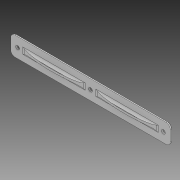
# Autodesk Inventor part: LEDLid
Saved by Autodesk Inventor 2020 (Build 240168000, 168)
## iProperties
Created: 2020-12-20
Part Number: LEDLid
Material: Generic
Document SubType Name: Modeling
Designer: DDeGo
Density: 1 g/cm^3
Appearance: Default
Author: DDeGo
Autodesk Inventor part; units mm, degrees
ref_plane "YZ Plane" through (0, 0, 0) normal (1, 0, 0) x (0, 1, 0)
ref_plane "XZ Plane" through (0, 0, 0) normal (0, 1, 0) x (-1, 0, 0)
ref_plane "XY Plane" through (0, 0, 0) normal (0, 0, 1) x (1, 0, 0)
sketch "Sketch1" plane through (0, 0, 0) normal (0, 0, 1) x (1, 0, 0)
  line L0 (71, -9) -> (-71, -9)
  line L1 (-75, -5) -> (-75, 5)
  line L2 (-71, 9) -> (71, 9)
  line L3 (75, 5) -> (75, -5)
  line L4 (75, -9) -> (-75, 9) construction
  line L5 (-75, -9) -> (75, 9) construction
  arc A0 (-71, 9) -> (-75, 5) centre (-71, 5) ccw
  arc A1 (-75, -5) -> (-71, -9) centre (-71, -5) ccw
  arc A2 (75, 5) -> (71, 9) centre (71, 5) ccw
  arc A3 (71, -9) -> (75, -5) centre (71, -5) ccw
  circle A4 centre (0, 0) radius 1.75
  line L6 (-75, 0) -> (-68.5, 0) construction
  line L7 (75, 0) -> (68.5, 0) construction
  circle A5 centre (-68.5, 0) radius 1.75
  circle A6 centre (68.5, 0) radius 1.75
  dimension "d0" = 4
  dimension "d2" = 150
  dimension "d3" = 18
  dimension "d4" = 3.5
  dimension "d5" = 6.5
  dimension "d6" = 6.5
  constraints: 16 end point, 8 point on circle, 8 point on line, 8 tangent, 7 centre point, 5 equal radius, 4 midpoint, 3 coincident, 3 horizontal, 2 parallel, 1 perpendicular
  measures "d0" radius of A0
  measures "d2" distance between parallel lines of L1 L3
  measures "d3" distance between parallel lines of L0 L2
  measures "d4" diameter of A4
  measures "d5" distance of L6.start L6.end
  measures "d6" distance of L7.start L7.end
extrude "Extrusion1" add sketch "Sketch1" along normal blind 1.5
sketch "Sketch2" plane through (0, 0, 0) normal (0, 1, 0) x (-1, 0, 0)
  line L0 (71, 1.5) -> (-71, 1.5) projected
  arc A0 (62.75, 1.5) -> (5.75, 1.5) centre (34.25, -159.7) ccw
  line L1 (-1.75, 1.5) -> (1.75, 1.5) projected
  line L2 (0, 1.5) -> (0, 8.4786) construction
  line L3 (66.75, 1.5) -> (70.25, 1.5) projected
  line L4 (66.75, 1.5) -> (62.75, 1.5) construction
  line L5 (5.75, 1.5) -> (1.75, 1.5) construction
  line L6 (1.75, 1.5) -> (1.75, 0) projected
  line L7 (46.1417, 4) -> (24.4242, 4) construction
  point P0 (0, 0)
  dimension "d9" = 4
  dimension "d10" = 2.5
  constraints: 8 end point, 2 horizontal, 2 point on circle, 1 centre point, 1 collinear, 1 midpoint, 1 perpendicular, 1 tangent, 1 vertical, 3 other
  measures "d9" distance of L4.end L3.start
extrude "Extrusion2" add sketch "Sketch2" along normal mid plane 2
fillet "Fillet1" radius 2 2 edges at (-34.25, -1, 1.5) (-34.25, 1, 1.5)
fillet "Fillet1" radius 10 2 edges at (-62.75, 0, 1.5) (-5.75, 0, 1.5)
mirror "Mirror1" about plane through (0, 0, 0) normal (1, 0, 0) of "Extrusion2", "Fillet1"
chamfer "Chamfer1" distance 0.5 angle 45 8 edges at (0, -9, 0) (73.8284, -7.8284, 0) (75, 0, 0) (73.8284, 7.8284, 0) (0, 9, 0) (-73.8284, 7.8284, 0) (-75, 0, 0) (-73.8284, -7.8284, 0)
body "Solid1"
